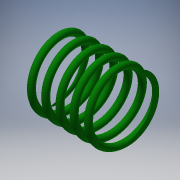
# Autodesk Inventor part: Component 23 (Valve Spring)
Saved by Autodesk Inventor 2018 (Build 220112000, 112)
## iProperties
Created: 2023-03-25
Part Number: Component 23 (Valve Spring)
Material: Generic
Document SubType Name: Modeling
Designer: Habib Mohamed
Density: 1 g/cm^3
Appearance: Dark Green
Author: Habib Mohamed
Autodesk Inventor part; units mm, degrees
ref_plane "YZ Plane" through (0, 0, 0) normal (1, 0, 0) x (0, 1, 0)
ref_plane "XZ Plane" through (0, 0, 0) normal (0, 1, 0) x (-1, 0, 0)
ref_plane "XY Plane" through (0, 0, 0) normal (0, 0, 1) x (1, 0, 0)
sketch "Sketch1" plane through (0, 0, 0) normal (0, 1, 0) x (-1, 0, 0)
  line L0 (0, 0) -> (3.9581, 0) construction
  circle A0 centre (0, 3.8) radius 0.4
  dimension "d0" = 0.8
  dimension "d1" = 3.8
  constraints: 2 end point, 1 centre point, 1 horizontal
  measures "d0" diameter of A0
  measures "d1" distance from line of L0 A0.centre
coil "Coil1" sketch "Sketch1" operation add axis through (0, 0, 0) along (-1, 0, 0) pitch 1.78 turns 9 hand right
sketch "Sketch2" plane through (0, 0, 0) normal (0, 1, 0) x (-1, 0, 0)
  line L0 (19.2726, 5.5) -> (12.2726, 5.5)
  line L1 (12.2726, 5.5) -> (12.2726, -5.5)
  line L2 (12.2726, -5.5) -> (19.2726, -5.5)
  line L3 (19.2726, -5.5) -> (19.2726, 5.5)
  line L4 (0.8726, 5.5) -> (-6.1274, 5.5)
  line L5 (-6.1274, 5.5) -> (-6.1274, -5.5)
  line L6 (-6.1274, -5.5) -> (0.8726, -5.5)
  line L7 (0.8726, -5.5) -> (0.8726, 5.5)
  line L8 (0, 0) -> (25.5435, 0) construction
  dimension "d10" = 11.4
  dimension "d11" = 7
  dimension "d12" = 11
  constraints: 18 end point, 4 parallel, 3 horizontal, 2 equal length, 2 perpendicular, 1 point on line, 1 other
  measures "d10" distance between parallel lines of L7 L1
  measures "d11" distance of L1.end L2.end
  measures "d12" distance of L2.end L0.start
extrude "Extrusion1" cut sketch "Sketch2" along normal mid plane 39.5
body "Solid1"
